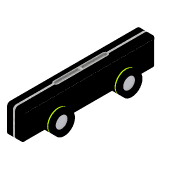
# Autodesk Inventor part: zedmini_camera
Saved by Autodesk Inventor 2017 (Build 210142000, 142)
## iProperties
Created: 2018-08-30
Part Number: zedmini_camera
Material: Generic
Document SubType Name: Modeling
Designer: ER2C
Density: 1 g/cm^3
Appearance: Default
Author: ER2C
Autodesk Inventor part; units mm, degrees
sketch "Sketch1" plane through (0, 0, 0) normal (0, 1, 0) x (-1, 0, 0)
  line L0 (6.5, -62.25) -> (-6.5, -62.25)
  line L1 (-6.5, -62.25) -> (-6.5, 62.25)
  line L2 (-6.5, 62.25) -> (6.5, 62.25)
  line L3 (6.5, 62.25) -> (6.5, -62.25)
  line L4 (6.5, -62.25) -> (-6.5, 62.25) construction
  line L5 (-6.5, -62.25) -> (6.5, 62.25) construction
  point P0 (0, 0)
  dimension "d0" = 13
  dimension "d1" = 124.5
  constraints: 12 end point, 2 midpoint, 2 parallel, 1 horizontal, 1 perpendicular
  measures "d0" distance of L1.end L2.end
  measures "d1" distance of L0.end L1.end
extrude "Extrusion1" add sketch "Sketch1" along normal mid plane 26.5
fillet "Fillet1" radius 3 4 edges at (0, 13.25, 62.25) (0, -13.25, 62.25) (0, -13.25, -62.25) (0, 13.25, -62.25)
ref_plane "Work Plane1" through (8.5, -10.25, 62.25) normal (1, 0, 0) x (0, 0, -1)
sketch "Sketch2" plane through (8.5, -10.25, 62.25) normal (1, 0, 0) x (0, 0, -1)
  arc A0 (122.5, 20.5) -> (121.5, 21.5) centre (121.5, 20.5) ccw
  line L0 (122.5, 20.5) -> (122.5, 0)
  arc A1 (121.5, -1) -> (122.5, 0) centre (121.5, 0) ccw
  line L1 (121.5, -1) -> (3, -1)
  arc A2 (2, 0) -> (3, -1) centre (3, 0) ccw
  line L2 (2, 0) -> (2, 20.5)
  arc A3 (3, 21.5) -> (2, 20.5) centre (3, 20.5) ccw
  line L3 (3, 21.5) -> (121.5, 21.5)
  constraints: 8 end point, 8 point on circle, 4 centre point
ref_plane "Work Plane2" through (8.5, -10.25, 60.25) normal (1, 0, 0) x (0, 0, -1)
sketch "Sketch3" plane through (8.5, -10.25, 60.25) normal (1, 0, 0) x (0, 0, -1)
  line L0 (-2, 20.5) -> (-2, 0) projected
  line L1 (-2, 10.25) -> (21, 10.25)
  circle A0 centre (21, 10.25) radius 10
  circle A1 centre (84, 10.25) radius 10
  point P0 (60.25, 10.25)
  dimension "d11" = 23
  dimension "d12" = 20
  dimension "d14" = 20
  dimension "d15" = 63
  constraints: 2 centre point, 2 end point, 1 coincident, 1 horizontal, 1 midpoint
  measures "d11" distance of L1.start L1.end
  measures "d12" diameter of A0
  measures "d14" diameter of A1
  measures "d15" distance of A1.centre L1.end
loft "Loft2" add profiles "Sketch2" section 1 edges at (6.5, 12.3713, -61.3713) (6.5, 13.25, 0) (6.5, 12.3713, 61.3713) (6.5, 0, 62.25) (6.5, -12.3713, 61.3713) (6.5, -13.25, 0) (6.5, -12.3713, -61.3713) (6.5, 0, -62.25)
extrude "Extrusion3" add sketch "Sketch3" along normal blind 15.5
ref_plane "Work Plane3" through (22, 0, 39.25) normal (1, 0, 0) x (0, 0, -1)
sketch "Sketch4" plane through (22, 0, 39.25) normal (1, 0, 0) x (0, 0, -1)
  circle A0 centre (0, 0) radius 6.5
  point P0 (39.25, 0)
  point P1 (63, 0)
  dimension "d26" = 13
  constraints: 1 centre point, 1 coincident
  measures "d26" diameter of A0
sketch "Sketch5" plane through (22, 0, 39.25) normal (1, 0, 0) x (0, 0, -1)
  circle A0 centre (0, 0) radius 6.5 projected
  point P0 (39.25, 0)
ref_plane "Work Plane4" through (21.5, 0, 39.25) normal (1, 0, 0) x (0, 0, -1)
sketch "Sketch6" plane through (21.5, 0, 39.25) normal (1, 0, 0) x (0, 0, -1)
  circle A0 centre (0, 0) radius 5.5
  point P0 (39.25, 0)
  dimension "d34" = 11
  constraints: 1 centre point
  measures "d34" diameter of A0
sketch "Sketch7" plane through (24, 0, 39.25) normal (1, 0, 0) x (0, 0, -1)
  circle A0 centre (0, 0) radius 9.75
  point P0 (39.25, 0)
  dimension "d37" = 19.5
  constraints: 1 centre point
  measures "d37" diameter of A0
loft "Loft4" cut profiles "Sketch7", "Sketch4"
extrude "Extrusion6" cut sketch "Sketch5" against normal blind 0.5
extrude "Extrusion7" cut sketch "Sketch6" against normal blind 0.5
sketch "Sketch8" plane through (0, 13.25, 0) normal (0, 1, 0) x (1, 0, 0)
  line L0 (24, -49.25) -> (24, -29.25) projected
  line L1 (24, -29.25) -> (19, -29.25)
  line L2 (19, 59.308) -> (18, 59.308)
  line L3 (18, 59.308) -> (18, -65.0875)
  line L4 (18, -65.0875) -> (19, -65.0875)
  line L5 (19, -65.0875) -> (19, 59.308)
  point P0 (0, 0)
  dimension "d46" = 5
  dimension "d47" = 1
  constraints: 10 end point, 2 horizontal, 2 parallel, 1 perpendicular
  measures "d46" distance of L0.end L1.end
  measures "d47" distance of L4.end L3.end
ref_plane "Work Plane5" through (-6.5, -10.25, 7.75) normal (0, 0, 1) x (1, 0, 0)
mirror "Mirror1" about plane through (-6.5, -10.25, 7.75) normal (0, 0, 1) of "Loft4", "Extrusion6", "Extrusion7"
split_face "Split2"
sketch "Sketch9" plane through (0, 13.25, 0) normal (0, 1, 0) x (1, 0, 0)
  line L0 (0, 0) -> (0, -1)
  line L1 (0, -1) -> (-1.25, -1)
  line L2 (0, -24.5) -> (0, -23)
  arc A0 (-1.5, -23) -> (1.5, -23) centre (0, -23) ccw
  line L3 (-1.5, -23) -> (-1.5, -1.25)
  line L4 (1.5, -23) -> (1.5, -1.25)
  line L5 (1.25, -1) -> (0, -1)
  arc A1 (-1.25, -1) -> (-1.5, -1.25) centre (-1.25, -1.25) ccw
  arc A2 (1.5, -1.25) -> (1.25, -1) centre (1.25, -1.25) ccw
  line L6 (0, 0) -> (0.625, 0)
  point P0 (-1.5, -1)
  dimension "d49" = 1
  dimension "d50" = 1.5
  dimension "d51" = 23.5
  dimension "d52" = 1.5
  dimension "d53" = 0.25
  constraints: 14 end point, 7 point on circle, 4 tangent, 3 centre point, 2 perpendicular, 2 point on line, 2 vertical, 1 coincident, 1 equal radius, 1 horizontal
  measures "d49" distance of L0.start L0.end
  measures "d50" distance of L0.end point (-1.5, -1)
  measures "d51" distance of L0.end L2.start
  measures "d52" distance of L2.start L2.end
  measures "d53" radius of A1
extrude "Extrusion8" cut sketch "Sketch9" against normal blind 2
sketch "Sketch10" plane through (0, 11.25, 0) normal (0, 1, 0) x (1, 0, 0)
  arc A0 (-1.5, -23) -> (1.5, -23) centre (0, -23) ccw projected
  circle A1 centre (0, -23) radius 0.75
  point P0 (0, 0)
  dimension "d56" = 1.5
  constraints: 1 centre point, 1 coincident
  measures "d56" diameter of A1
extrude "Extrusion9" cut sketch "Sketch10" against normal blind 1
mirror "Mirror2" about plane through (0, 0, 0) normal (0, 0, 1) of "Extrusion8", "Extrusion9"
ref_plane "Work Plane6" through (0, 16.25, 0) normal (0, 1, 0) x (1, 0, 0)
sketch "Sketch11" plane through (0, 16.25, 0) normal (0, 1, 0) x (1, 0, 0)
  arc A0 (-1.5, -23) -> (1.5, -23) centre (0, -23) ccw projected
  arc A1 (1.5, 23) -> (-1.5, 23) centre (0, 23) ccw projected
  line L0 (0, 23) -> (0, -23) construction
  line L1 (-2.5, 23) -> (-2.5, -23)
  line L2 (2.5, -23) -> (2.5, 23)
  line L3 (0, -23) -> (-1, -23)
  line L4 (1, -25.2913) -> (1, -100.0125)
  line L5 (1, -100.0125) -> (-1, -100.0125)
  line L6 (-1, -100.0125) -> (-1, -25.2913)
  arc A2 (-2.5, -23) -> (-1, -25.2913) centre (0, -23) ccw
  arc A3 (1, -25.2913) -> (2.5, -23) centre (0, -23) ccw
  line L7 (1, 25.2913) -> (1, 101.6)
  line L8 (1, 101.6) -> (-1, 101.6)
  line L9 (-1, 101.6) -> (-1, 25.2913)
  arc A4 (2.5, 23) -> (1, 25.2913) centre (0, 23) ccw
  arc A5 (-1, 25.2913) -> (-2.5, 23) centre (0, 23) ccw
  circle A6 centre (0, -23) radius 0.75 projected
  line L10 (-1.25, -1) -> (1.25, -1) projected
  arc A7 (-1.25, -1) -> (-1.5, -1.25) centre (-1.25, -1.25) ccw projected
  line L11 (-1.5, -23) -> (-1.5, -1.25) projected
  arc A8 (-1.5, -23) -> (1.5, -23) centre (0, -23) ccw projected
  line L12 (1.5, -1.25) -> (1.5, -23) projected
  arc A9 (1.5, -1.25) -> (1.25, -1) centre (1.25, -1.25) ccw projected
  circle A10 centre (0, 23) radius 0.75 projected
  line L13 (-1.25, 1) -> (1.25, 1) projected
  arc A11 (1.25, 1) -> (1.5, 1.25) centre (1.25, 1.25) ccw projected
  line L14 (1.5, 1.25) -> (1.5, 23) projected
  arc A12 (1.5, 23) -> (-1.5, 23) centre (0, 23) ccw projected
  line L15 (-1.5, 23) -> (-1.5, 1.25) projected
  arc A13 (-1.5, 1.25) -> (-1.25, 1) centre (-1.25, 1.25) ccw projected
  point P0 (0, 0)
  dimension "d61" = 1
  dimension "d62" = 2
  constraints: 22 end point, 8 point on circle, 4 centre point, 4 tangent, 3 parallel, 1 horizontal, 1 midpoint, 1 vertical
  measures "d61" distance of L0.end L3.end
  measures "d62" distance of L4.end L5.end
sketch "Sketch12" plane through (0, -13.25, 0) normal (0, -1, 0) x (1, 0, 0)
  line L0 (-1.5, -1.25) -> (-1.5, -23)
  arc A0 (-1.5, -23) -> (1.5, -23) centre (0, -23) ccw
  line L1 (1.5, -23) -> (1.5, -1.25)
  line L2 (1.5, 1.25) -> (1.5, 23)
  arc A1 (1.5, 23) -> (-1.5, 23) centre (0, 23) ccw
  line L3 (-1.5, 23) -> (-1.5, 1.25)
  line L4 (-6.5, -59.25) -> (6.5, -59.25) projected
  line L5 (-6.5, -59.25) -> (-6.5, 59.25) projected
  line L6 (6.5, 59.25) -> (-6.5, 59.25) projected
  line L7 (6.5, 59.25) -> (6.5, -59.25) projected
  line L8 (0, -23) -> (0, 23) construction
  line L9 (-1.5, -23) -> (-1.5, 23)
  line L10 (1.5, 23) -> (1.5, -23)
  arc A2 (-1.5, -23) -> (1.5, -23) centre (0, -23) ccw
  arc A3 (1.5, 23) -> (-1.5, 23) centre (0, 23) ccw
  constraints: 16 end point, 8 point on circle, 5 centre point
extrude "Extrusion10" cut sketch "Sketch12" against normal blind 2 contours L9 L3 A1 L2 L10 L1 A0 L0
sketch "Sketch13" plane through (0, -11.25, 0) normal (0, -1, 0) x (1, 0, 0)
  circle A0 centre (0, -23) radius 0.75 projected
  circle A1 centre (0, 23) radius 0.75 projected
  point P0 (0, 0)
extrude "Extrusion11" cut sketch "Sketch13" against normal blind 1
split_face "Split3"
sketch "Sketch14" plane through (8.5, -10.25, 60.25) normal (1, 0, 0) x (0, 0, -1)
  arc A0 (1, 21.5) -> (0, 20.5) centre (1, 20.5) ccw projected
  line L0 (119.5, 21.5) -> (1, 21.5) projected
  circle A1 centre (21, 10.25) radius 10 projected
  circle A2 centre (84, 10.25) radius 10 projected
  arc A3 (120.5, 20.5) -> (119.5, 21.5) centre (119.5, 20.5) ccw projected
  line L1 (119.5, 21.5) -> (1, 21.5) projected
  arc A4 (1, 21.5) -> (0, 20.5) centre (1, 20.5) ccw projected
  line L2 (0, 20.5) -> (0, 0) projected
  arc A5 (0, 0) -> (1, -1) centre (1, 0) ccw projected
  line L3 (1, -1) -> (119.5, -1) projected
  arc A6 (119.5, -1) -> (120.5, 0) centre (119.5, 0) ccw projected
  line L4 (120.5, 0) -> (120.5, 20.5) projected
  arc A7 (1, 21.4) -> (0.1, 20.5) centre (1, 20.5) ccw
  arc A8 (0.1, 0) -> (1, -0.9) centre (1, 0) ccw
  arc A9 (120.4, 20.5) -> (119.5, 21.4) centre (119.5, 20.5) ccw
  arc A10 (119.5, -0.9) -> (120.4, 0) centre (119.5, 0) ccw
  line L5 (1, 21.4) -> (119.5, 21.4)
  line L6 (120.4, 20.5) -> (120.4, 0)
  line L7 (119.5, -0.9) -> (1, -0.9)
  line L8 (0.1, 0) -> (0.1, 20.5)
  point P0 (60.25, 10.25)
  dimension "d67" = 1.8
  dimension "d68" = 1.8
  dimension "d69" = 1.8
  dimension "d70" = 1.8
  constraints: 8 end point, 8 point on circle, 5 tangent, 4 centre point, 4 coincident, 1 perpendicular
  measures "d67" diameter of A7
  measures "d68" diameter of A8
  measures "d69" diameter of A9
  measures "d70" diameter of A10
extrude "Extrusion12" cut sketch "Sketch14" against normal blind 0.25 contours L0 A3 L4 A6 L3 A5 L2 A0
body "Solid1"
